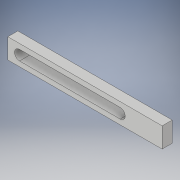
# Autodesk Inventor part: creat3
Saved by Autodesk Inventor 2019 (Build 230136000, 136)
## iProperties
Created: 2021-11-12
Part Number: creat3
Material: 一般
Document SubType Name: Sheet Metal
Designer: yuta
Density: 1 g/cm^3
Sheet Metal Rule: Default_mm
Appearance: 既定
Author: yuta
Autodesk Inventor part; units mm, degrees
ref_plane "YZ Plane" through (0, 0, 0) normal (1, 0, 0) x (0, 1, 0)
ref_plane "XZ Plane" through (0, 0, 0) normal (0, 1, 0) x (-1, 0, 0)
ref_plane "XY Plane" through (0, 0, 0) normal (0, 0, 1) x (1, 0, 0)
sketch "スケッチ1" plane through (0, 0, 0) normal (0, 0, 1) x (1, 0, 0)
  line L0 (-25.7132, 3.9746) -> (20.2868, 3.9746)
  line L1 (20.2868, 3.9746) -> (20.2868, -2.0254)
  line L2 (20.2868, -2.0254) -> (-25.7132, -2.0254)
  line L3 (-25.7132, -2.0254) -> (-25.7132, 3.9746)
  point P0 (0, 0)
  dimension "d0" = 46
  dimension "d1" = 6
  constraints: 8 end point, 2 parallel, 1 horizontal, 1 perpendicular
  measures "d0" distance of L1.end L2.end
  measures "d1" distance of L0.end L1.end
extrude "押し出し1" add sketch "スケッチ1" along normal blind 3
sketch "スケッチ2" plane through (0, 0, 3) normal (0, 0, 1) x (1, 0, 0)
  line L0 (-22.2132, 0.9746) -> (7.7868, 0.9746) construction
  line L1 (-22.2132, -0.5254) -> (7.7868, -0.5254)
  line L2 (7.7868, 2.4746) -> (-22.2132, 2.4746)
  arc A0 (-22.2132, 2.4746) -> (-22.2132, -0.5254) centre (-22.2132, 0.9746) ccw
  arc A1 (7.7868, -0.5254) -> (7.7868, 2.4746) centre (7.7868, 0.9746) ccw
  line L3 (-25.7132, 3.9746) -> (-25.7132, -2.0254) projected
  line L4 (20.2868, 3.9746) -> (-25.7132, 3.9746) projected
  point P0 (0, 0)
  point P1 (-7.2132, 0.9746)
  dimension "d4" = 30
  dimension "d5" = 3
  dimension "d6" = 3.5
  dimension "d7" = 3
  constraints: 8 end point, 4 point on circle, 4 tangent, 2 centre point, 1 horizontal, 1 midpoint, 1 parallel
  measures "d4" distance of L0.start L0.end
  measures "d5" diameter of A1
  measures "d6" distance from line of L3 L0.start
  measures "d7" distance from line of L4 L0.start
extrude "押し出し2" cut sketch "スケッチ2" against normal blind 3
equation "\"BendRadius\" = Thickness"
equation "\"BendReliefWidth\" = Thickness"
equation "\"BendReliefDepth\" = 0.5 * Thickness"
equation "\"CornerReliefSize\" = 4 * Thickness"
equation "\"MinimumRemnant\" = 2 * Thickness"
equation "\"TransitionRadius\" = BendRadius"
equation "\"JacobiRadiusSize\" = BendRadius"
equation "\"GapSize\" = Thickness"
equation "\"Thickness\" = 0.5"
